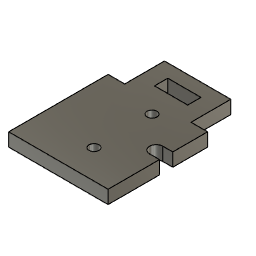
Holder pogonskih motora (Autodesk Fusion 360 design; units mm, degrees)
Autodesk Fusion 360 part; units mm, degrees
note: some values were not read from the file. Set by a fixed rule: which sketch regions a step uses.
sketch "Sketch1" plane through (0, 0, 0) normal (0, 0, 1) x (1, 0, 0)
  line L0 (15, -15) -> (-15, -15)
  line L1 (-15, -15) -> (-15, 15)
  line L2 (-10, 15) -> (-10, 27)
  line L3 (-10, 27) -> (10, 27)
  line L4 (10, 27) -> (10, 15)
  line L5 (-5, 19) -> (-5, 23)
  line L6 (-5, 23) -> (5, 23)
  line L7 (5, 23) -> (5, 19)
  line L8 (-15, 15) -> (-10, 15)
  line L9 (10, 15) -> (15, 15)
  line L10 (0, 70) -> (0, -30) construction
  line L11 (15, 0.5) -> (12, 0.5)
  line L12 (12, 4.5) -> (15, 4.5)
  arc A0 (12, 4.5) -> (12, 0.5) centre (12, 2.5) ccw
  line L13 (15, 15) -> (15, 4.5)
  line L14 (15, 0.5) -> (15, -15)
  circle A1 centre (2, 11.25) radius 1.5
  circle A2 centre (2, -6.25) radius 1.5
  line L15 (-5, 19) -> (5, 19)
  dimension "d1" = 30
  dimension "d3" = 12
  dimension "d4" = 20
  dimension "d7" = 4
  dimension "d8" = 10
  dimension "d9" = 42
  dimension "d17" = 12.5
  dimension "d18" = 2
  dimension "d21" = 17.5
  dimension "d22" = 3
  dimension "d23" = 3
  dimension "d24" = 10
  dimension "d25" = 3
  dimension "d29" = 4
  constraint horizontal L0
  constraint perpendicular L0 L1
  constraint parallel L0 L8
  constraint parallel L1 L13
  constraint perpendicular L2 L3
  constraint coincident L4.end L8
  constraint perpendicular L4 L8
  constraint perpendicular L3 L5
  constraint perpendicular L5 L6
  constraint perpendicular L6 L7
  constraint collinear L8 L9
  constraint vertical L10
  constraint perpendicular L11 L13
  constraint collinear L13 L14
  measures "d1" distance of L1.end L9.end
  measures "d3" distance of L2.start L2.end
  measures "d4" distance of L2.end L3.end
  measures "d7" distance of L5.start L5.end
  measures "d8" distance of L5.end L6.end
  measures "d9" distance of L0 L3
  measures "d17" distance of L9 A0.centre
  measures "d18" radius of A0
  measures "d21" distance of A1.centre A2.centre
  measures "d22" diameter of A1
  measures "d23" diameter of A2
  measures "d24" horizontal distance of A0.centre A2.centre
  measures "d25" distance of A0.centre L14
  measures "d29" distance of L9 L15
extrude "Extrude1" add sketch "Sketch1" along normal blind 4
